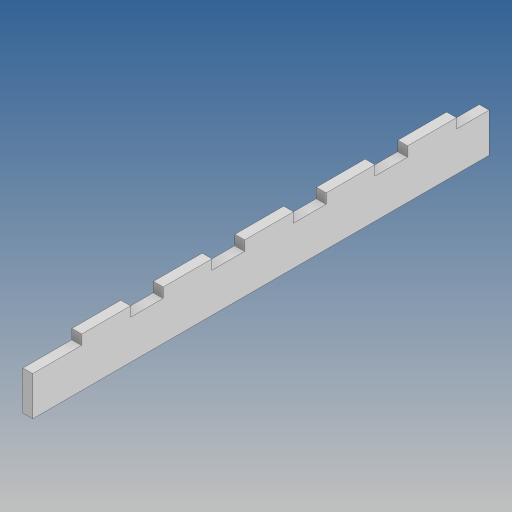
# Autodesk Inventor part: Pieza3
Saved by Autodesk Inventor 2024 (Build 280153000, 153)
## iProperties
Created: 2024-05-31
Part Number: Pieza3
Material: Genérico
Document SubType Name: Modeling
Designer: Pablo
Density: 1 g/cm^3
Appearance: Valor por defecto
Author: Pablo
Autodesk Inventor part; units mm, degrees
ref_plane "YZ Plane" through (0, 0, 0) normal (1, 0, 0) x (0, 1, 0)
ref_plane "XZ Plane" through (0, 0, 0) normal (0, 1, 0) x (-1, 0, 0)
ref_plane "XY Plane" through (0, 0, 0) normal (0, 0, 1) x (1, 0, 0)
sketch "Boceto1" plane through (0, 0, 0) normal (1, 0, 0) x (0, 1, 0)
  line L0 (0, 0) -> (12, 0)
  line L1 (12, 0) -> (12, -140)
  line L2 (12, -140) -> (0, -140)
  line L3 (0, -140) -> (0, 0)
  line L4 (12, -15) -> (15, -15)
  line L5 (15, -15) -> (15, -30)
  line L6 (15, -30) -> (12, -30)
  line L7 (12, -30) -> (12, -15)
  line L8 (12, -40) -> (15, -40)
  line L9 (15, -40) -> (15, -55)
  line L10 (15, -55) -> (12, -55)
  line L11 (12, -55) -> (12, -40)
  line L12 (12, -65) -> (15, -65)
  line L13 (15, -65) -> (15, -80)
  line L14 (15, -80) -> (12, -80)
  line L15 (12, -80) -> (12, -65)
  line L16 (12, -90) -> (15, -90)
  line L17 (15, -90) -> (15, -105)
  line L18 (15, -105) -> (12, -105)
  line L19 (12, -105) -> (12, -90)
  line L20 (12, -115) -> (15, -115)
  line L21 (15, -115) -> (15, -130)
  line L22 (15, -130) -> (12, -130)
  line L23 (12, -130) -> (12, -115)
  point P0 (12, -130)
  point P1 (12, -115)
  point P2 (12, -105)
  point P3 (12, -90)
  point P4 (12, -65)
  point P5 (12, -55)
  point P6 (12, -40)
  dimension "d0" = 12
  dimension "d1" = 140
  dimension "d5" = 3
  dimension "d6" = 15
  dimension "d7" = 15
  dimension "d10" = 25
  constraints: 48 end point, 4 parallel, 2 horizontal, 2 perpendicular, 1 point on line, 1 vertical, 32 other
  measures "d0" distance of L1.end L2.end
  measures "d1" distance of L0.end L1.end
  measures "d5" distance of L5.end L6.end
  measures "d6" distance of L4.end L5.end
  measures "d7" distance between parallel lines of L4 L0
  measures "d10" distance of L4.start L8.start
extrude "Extrusión1" add sketch "Boceto1" along normal blind 3
